Autodesk Inventor part; units mm, degrees
(part 4 of 5)
sketch "Sketch9" plane through (0, 0, -3) normal (0, 0, -1) x (-1, 0, 0)
  line L0 (143, 0.6) -> (143, 11.3716)
  line L1 (157, 15.8) -> (157, 15.2)
  line L2 (157, 15.2) -> (155.0929, 13.2929)
  line L3 (143.6142, 13) -> (154.3858, 13)
  line L4 (142.9071, 13.2929) -> (141, 15.2)
  line L5 (143.6142, 18) -> (154.3858, 18)
  line L6 (154.3858, 13) -> (143.6142, 13)
  line L7 (126.6142, 18) -> (137.3858, 18)
  line L8 (143, 11.3716) -> (143, 0.6)
  line L9 (138, 0.6) -> (138, 11.3716)
  line L10 (143, -5.6284) -> (143, -16.4)
  line L11 (138, -16.4) -> (138, -5.6284)
  line L12 (157, 15.8) -> (155.0929, 17.7071) projected
  line L13 (155.0929, 17.7071) -> (157, 15.8)
  line L14 (157, 15.2) -> (157, 15.8) projected
  line L15 (157, 15.8) -> (157, 15.2)
  line L16 (157, 15.2) -> (155.0929, 13.2929)
  line L17 (141, 15.8) -> (140, 15.8)
  line L18 (140, 15.8) -> (138.0929, 17.7071)
  line L19 (138.0929, 17.7071) -> (140, 15.8) projected
  line L20 (140.2, 13.9858) -> (140.2, 15.2)
  line L21 (140.2, 15.2) -> (140, 15.2)
  line L22 (138.2929, 12.0787) -> (140.2, 13.9858)
  line L23 (140.2, -2.0142) -> (138.2929, -0.1071) projected
  line L24 (138.2929, -0.1071) -> (140.2, -2.0142)
  line L25 (140.2, -2.0142) -> (140.2, -3.0142)
  line L26 (140.2, -3.0142) -> (138.2929, -4.9213)
  line L27 (138.2929, -17.1071) -> (140.2, -19.0142)
  line L28 (140.2, -19.0142) -> (140.8, -19.0142)
  line L29 (143, -16.4) -> (143, -5.6284)
  line L30 (140.8, -3.0142) -> (142.7071, -4.9213) projected
  line L31 (142.7071, -4.9213) -> (140.8, -3.0142)
  line L32 (140.8, -3.0142) -> (140.8, -2.0142)
  line L33 (142.7071, -0.1071) -> (140.8, -2.0142)
  line L34 (142.7071, 12.0787) -> (140.8, 13.9858)
  line L35 (140.8, 15.2) -> (141, 15.2)
  line L36 (140.8, 15.2) -> (140.8, 13.9858)
  line L37 (111.2, 0.5) -> (109.2929, 2.4071) projected
  line L38 (111.8, 16.5) -> (113.7071, 14.5929) projected
  line L39 (113.7071, 14.5929) -> (111.8, 16.5)
  line L40 (111.8, 16.5) -> (111.2, 16.5) projected
  line L41 (111.8, 16.5) -> (111.2, 16.5)
  line L42 (111.2, 16.5) -> (109.2929, 14.5929)
  line L43 (94.5, -0.2) -> (96.4071, 1.7071) projected
  line L44 (96.4071, 1.7071) -> (94.5, -0.2)
  line L45 (94.5, -0.2) -> (94.5, -0.8) projected
  line L46 (94.5, -0.2) -> (94.5, -0.8)
  line L47 (94.5, -0.8) -> (96.4071, -2.7071)
  line L48 (109.2929, -15.5929) -> (111.2, -17.5) projected
  line L49 (109.2929, -15.5929) -> (111.2, -17.5)
  line L50 (111.8, -17.5) -> (111.2, -17.5) projected
  line L51 (111.2, -17.5) -> (111.8, -17.5)
  line L52 (111.8, -17.5) -> (113.7071, -15.5929)
  line L53 (126.5929, -2.7071) -> (128.5, -0.8)
  line L54 (128.5, -0.2) -> (126.5929, 1.7071)
  line L55 (140.8, -19.0142) -> (140.2, -19.0142) projected
  line L56 (140.8, -19.0142) -> (142.7071, -17.1071)
  line L57 (140, 15.2) -> (138.0929, 13.2929)
  line L58 (125.9071, 13.2929) -> (124, 15.2)
  line L59 (124, 15.2) -> (124, 15.8)
  line L60 (124, 15.8) -> (125.9071, 17.7071)
  line L61 (126.6142, 18) -> (137.3858, 18)
  line L62 (126.6142, 13) -> (137.3858, 13)
  line L63 (110.5, -0.2) -> (108.75, 1.55)
  line L64 (108.5929, 1.7071) -> (110.5, -0.2) projected
  line L65 (108.5929, -2.7071) -> (110.5, -0.8) projected
  line L66 (110.5, -0.8) -> (108.5929, -2.7071)
  line L67 (110.5, -0.2) -> (108.5929, 1.7071)
  line L68 (113.7071, 2.4071) -> (111.8, 0.5) projected
  line L69 (111.8, 0.5) -> (113.7071, 2.4071)
  line L70 (112.5, -0.2) -> (114.4071, 1.7071) projected
  line L71 (112.5, -0.2) -> (114.4071, 1.7071)
  line L72 (112.5, -0.8) -> (114.4071, -2.7071)
  line L73 (109.2929, -3.4071) -> (111.2, -1.5) projected
  line L74 (111.2, -1.5) -> (109.2929, -3.4071)
  line L75 (111.8, -1.5) -> (113.7071, -3.4071)
  line L76 (113.7071, -3.4071) -> (111.8, -1.5) projected
  line L77 (111.2, 0.5) -> (109.2929, 2.4071)
  line L78 (111.2, -1.5) -> (111.2, -0.8)
  line L79 (111.2, -0.2) -> (111.2, 0.5)
  line L80 (110.5, -0.2) -> (111.2, -0.2)
  line L81 (111.8, -0.2) -> (112.5, -0.2)
  line L82 (111.8, 0.5) -> (111.8, -0.2)
  line L83 (111.8, -0.8) -> (111.8, -1.5)
  line L84 (112.5, -0.8) -> (111.8, -0.8)
  line L85 (111.2, -0.8) -> (110.5, -0.8)
  line L86 (97.1142, 2) -> (107.8858, 2)
  line L87 (109, 3.1142) -> (109, 13.8858)
  line L88 (109, -14.8858) -> (109, -4.1142)
  line L89 (107.8858, -3) -> (97.1142, -3)
  line L90 (114, -4.1142) -> (114, -14.8858)
  line L91 (125.8858, -3) -> (115.1142, -3)
  line L92 (114, 13.8858) -> (114, 3.1142)
  line L93 (115.1142, 2) -> (125.8858, 2)
  line L94 (-140, -35) -> (140, -35) projected
  line L95 (141, 15.8) -> (142.9071, 17.7071)
  line L96 (128.5, -0.2) -> (128.5, -0.8)
  line L97 (63.7142, 27) -> (80.4858, 27) projected
  line L98 (26.4142, 27) -> (43.1858, 27) projected
  line L99 (-20.3858, 27) -> (-3.6142, 27) projected
  line L100 (-57.6858, 27) -> (-40.9142, 27) projected
  line L101 (-104.4858, 27) -> (-87.7142, 27) projected
  line L102 (-141.7858, 27) -> (-125.0142, 27) projected
  line L103 (87, 20.4858) -> (87, 3.7142) projected
  line L104 (49.7, 20.4858) -> (49.7, 3.7142) projected
  line L105 (2.9, 20.4858) -> (2.9, 3.7142) projected
  line L106 (-34.4, 20.4858) -> (-34.4, 3.7142) projected
  line L107 (-81.2, 20.4858) -> (-81.2, 3.7142) projected
  line L108 (-118.5, 20.4858) -> (-118.5, 3.7142) projected
  line L109 (8.9, 9) -> (10.9, 11) projected
  line L110 (11.9, 11) -> (13.9, 9) projected
  line L111 (11.9, -9) -> (13.9, -11) projected
  line L112 (8.9, -11) -> (10.9, -9) projected
  line L113 (-72.2, 11) -> (-70.2, 9) projected
  line L114 (-70.2, 8) -> (-72.2, 6) projected
  line L115 (-72.2, -9) -> (-70.2, -11) projected
  line L116 (-75.2, -11) -> (-73.2, -9) projected
  arc A0 (109.2929, 14.5929) -> (109, 13.8858) centre (110, 13.8858) ccw
  arc A1 (114, 13.8858) -> (113.7071, 14.5929) centre (113, 13.8858) ccw
  arc A2 (113.7071, 2.4071) -> (114, 3.1142) centre (113, 3.1142) ccw
  arc A3 (109, 3.1142) -> (109.2929, 2.4071) centre (110, 3.1142) ccw
  arc A4 (108.5929, 1.7071) -> (107.8858, 2) centre (107.8858, 1) ccw
  arc A5 (115.1142, 2) -> (114.4071, 1.7071) centre (115.1142, 1) ccw
  arc A6 (114.4071, -2.7071) -> (115.1142, -3) centre (115.1142, -2) ccw
  arc A7 (114, -4.1142) -> (113.7071, -3.4071) centre (113, -4.1142) ccw
  arc A8 (109.2929, -3.4071) -> (109, -4.1142) centre (110, -4.1142) ccw
  arc A9 (107.8858, -3) -> (108.5929, -2.7071) centre (107.8858, -2) ccw
  arc A10 (97.1142, 2) -> (96.4071, 1.7071) centre (97.1142, 1) ccw
  arc A11 (96.4071, -2.7071) -> (97.1142, -3) centre (97.1142, -2) ccw
  arc A12 (109, -14.8858) -> (109.2929, -15.5929) centre (110, -14.8858) ccw
  arc A13 (113.7071, -15.5929) -> (114, -14.8858) centre (113, -14.8858) ccw
  arc A14 (125.8858, -3) -> (126.5929, -2.7071) centre (125.8858, -2) ccw
  arc A15 (126.5929, 1.7071) -> (125.8858, 2) centre (125.8858, 1) ccw
  arc A16 (138.0929, 17.7071) -> (137.3858, 18) centre (137.3858, 17) ccw
  arc A17 (126.6142, 18) -> (125.9071, 17.7071) centre (126.6142, 17) ccw
  arc A18 (125.9071, 13.2929) -> (126.6142, 13) centre (126.6142, 14) ccw
  arc A19 (137.3858, 13) -> (138.0929, 13.2929) centre (137.3858, 14) ccw
  arc A20 (138.2929, 12.0787) -> (138, 11.3716) centre (139, 11.3716) ccw
  arc A21 (143, 11.3716) -> (142.7071, 12.0787) centre (142, 11.3716) ccw
  arc A22 (142.9071, 13.2929) -> (143.6142, 13) centre (143.6142, 14) ccw
  arc A23 (143.6142, 18) -> (142.9071, 17.7071) centre (143.6142, 17) ccw
  arc A24 (155.0929, 17.7071) -> (154.3858, 18) centre (154.3858, 17) ccw
  arc A25 (154.3858, 13) -> (155.0929, 13.2929) centre (154.3858, 14) ccw
  arc A26 (154.3858, 13) -> (155.0929, 13.2929) centre (154.3858, 14) ccw
  arc A27 (138, 0.6) -> (138.2929, -0.1071) centre (139, 0.6) ccw
  arc A28 (142.7071, -0.1071) -> (143, 0.6) centre (142, 0.6) ccw
  arc A29 (143, -5.6284) -> (142.7071, -4.9213) centre (142, -5.6284) ccw
  arc A30 (138.2929, -4.9213) -> (138, -5.6284) centre (139, -5.6284) ccw
  arc A31 (138, -16.4) -> (138.2929, -17.1071) centre (139, -16.4) ccw
  arc A32 (142.7071, -17.1071) -> (143, -16.4) centre (142, -16.4) ccw
  line L117 (-58.3929, 1.9071) -> (-60.3, 0)
  line L118 (-39.1071, 3.0071) -> (-37.2, 1.1)
  line L119 (-38.3, 0) -> (-40.2071, 1.9071)
  line L120 (-40.2071, -2.5071) -> (-38.3, -0.6)
  line L121 (-38.3, -0.6) -> (-38.3, 0)
  line L122 (-38.3, 0) -> (-40.5, 2.2)
  line L123 (-40.2071, -22.8929) -> (-38.3, -24.8)
  line L124 (-39.1071, -21.7929) -> (-37.2, -23.7)
  line L125 (-59.4929, -21.7929) -> (-61.4, -23.7)
  line L126 (-58.3929, -22.8929) -> (-60.3, -24.8)
  line L127 (-38.3, 24.2) -> (-38.3, 24.8)
  line L128 (-58.3929, 26.7071) -> (-60.3, 24.8)
  line L129 (-60.3, 24.8) -> (-60.3, 24.2)
  line L130 (-60.3, 24.2) -> (-60.3, 24.8)
  line L131 (-58.3929, 22.2929) -> (-60.3, 24.2)
  line L132 (-59.4929, 21.1929) -> (-61.4, 23.1)
  line L133 (-62, 23.1) -> (-63.9071, 21.1929)
  line L134 (-63.9071, 3.0071) -> (-62, 1.1)
  line L135 (-62, 1.1) -> (-61.4, 1.1)
  line L136 (-61.4, 1.1) -> (-59.4929, 3.0071)
  line L137 (-59.4929, -3.6071) -> (-61.4, -1.7)
  line L138 (-62, -1.7) -> (-63.9071, -3.6071)
  line L139 (-64.2, -4.3142) -> (-64.2, -21.0858)
  line L140 (-63.9071, -21.7929) -> (-62, -23.7)
  line L141 (-60.3, -24.8) -> (-60.3, -25.4)
  line L142 (-60.3, -25.4) -> (-58.3929, -27.3071)
  line L143 (-57.6858, -27.6) -> (-40.9142, -27.6)
  line L144 (-40.2071, -27.3071) -> (-38.3, -25.4)
  line L145 (-38.3, -25.4) -> (-38.3, -24.8)
  line L146 (-37.2, -23.7) -> (-36.6, -23.7)
  line L147 (-36.6, -23.7) -> (-34.6929, -21.7929)
  line L148 (-34.4, -21.0858) -> (-34.4, -4.3142)
  line L149 (-34.6929, -3.6071) -> (-36.6, -1.7)
  line L150 (-36.6, -1.7) -> (-37.2, -1.7)
  line L151 (-37.2, -1.7) -> (-39.1071, -3.6071)
  line L152 (-38.3, -0.6) -> (-38.3, 0)
  line L153 (-36.6, 1.1) -> (-34.6929, 3.0071)
  line L154 (-34.4, 3.7142) -> (-34.4, 20.4858)
  line L155 (-34.6929, 21.1929) -> (-36.6, 23.1)
  line L156 (-36.6, 23.1) -> (-37.2, 23.1)
  line L157 (-37.2, 23.1) -> (-39.1071, 21.1929)
  line L158 (-38.3, 24.2) -> (-38.3, 24.8)
  line L159 (-57.6858, 27) -> (-40.9142, 27)
  line L160 (-64.2, 20.4858) -> (-64.2, 3.7142)
  line L161 (-38.3, 24.8) -> (-40.2071, 26.7071)
  line L162 (-38.3, 24.2) -> (-40.2071, 22.2929)
  line L163 (-37.2, 1.1) -> (-36.6, 1.1)
  arc A33 (-63.9071, 21.1929) -> (-64.2, 20.4858) centre (-63.2, 20.4858) ccw
  arc A34 (-57.6858, 27) -> (-58.3929, 26.7071) centre (-57.6858, 26) ccw
  arc A35 (-40.2071, 26.7071) -> (-40.9142, 27) centre (-40.9142, 26) ccw
  arc A36 (-34.4, 20.4858) -> (-34.6929, 21.1929) centre (-35.4, 20.4858) ccw
  arc A37 (-34.6929, 3.0071) -> (-34.4, 3.7142) centre (-35.4, 3.7142) ccw
  arc A38 (-34.4, -4.3142) -> (-34.6929, -3.6071) centre (-35.4, -4.3142) ccw
  arc A39 (-34.6929, -21.7929) -> (-34.4, -21.0858) centre (-35.4, -21.0858) ccw
  arc A40 (-40.9142, -27.6) -> (-40.2071, -27.3071) centre (-40.9142, -26.6) ccw
  arc A41 (-58.3929, -27.3071) -> (-57.6858, -27.6) centre (-57.6858, -26.6) ccw
  arc A42 (-64.2, -21.0858) -> (-63.9071, -21.7929) centre (-63.2, -21.0858) ccw
  arc A43 (-63.9071, -3.6071) -> (-64.2, -4.3142) centre (-63.2, -4.3142) ccw
  arc A44 (-64.2, 3.7142) -> (-63.9071, 3.0071) centre (-63.2, 3.7142) ccw
  line L164 (-62, 23.1) -> (-61.4, 23.1)
  line L165 (-60.3, 0) -> (-60.3, -0.6)
  line L166 (-58.3929, -2.5071) -> (-60.3, -0.6)
  line L167 (-62, -1.7) -> (-61.4, -1.7)
  line L168 (-62, -23.7) -> (-61.4, -23.7)
  line L169 (-57.1, 20.9) -> (-41.5, 20.9)
  line L170 (-39.4, 20.4858) -> (-39.4, 3.7142)
  line L171 (-41.5, 3.3) -> (-57.1, 3.3)
  line L172 (-59.2, 3.7142) -> (-59.2, 20.4858)
  line L173 (-57.6858, 22) -> (-40.9142, 22)
  line L174 (-40.5, 19.9) -> (-40.5, 4.3)
  line L175 (-40.9142, 2.2) -> (-57.6858, 2.2)
  line L176 (-58.1, 4.3) -> (-58.1, 19.9)
  line L177 (-57.1, -3.9) -> (-41.5, -3.9)
  line L178 (-39.4, -4.3142) -> (-39.4, -21.0858)
  line L179 (-41.5, -21.5) -> (-57.1, -21.5)
  line L180 (-59.2, -21.0858) -> (-59.2, -4.3142)
  line L181 (-57.6858, -22.6) -> (-40.9142, -22.6)
  line L182 (-40.5, -20.5) -> (-40.5, -4.9)
  line L183 (-40.9142, -2.8) -> (-57.6858, -2.8)
  line L184 (-58.1, -4.9) -> (-58.1, -20.5)
  arc A45 (-39.1071, 21.1929) -> (-39.4, 20.4858) centre (-38.4, 20.4858) ccw
  arc A46 (-40.9142, 22) -> (-40.2071, 22.2929) centre (-40.9142, 23) ccw
  arc A47 (-58.3929, 22.2929) -> (-57.6858, 22) centre (-57.6858, 23) ccw
  arc A48 (-59.2, 20.4858) -> (-59.4929, 21.1929) centre (-60.2, 20.4858) ccw
  arc A49 (-39.4, 3.7142) -> (-39.1071, 3.0071) centre (-38.4, 3.7142) ccw
  arc A50 (-39.1071, -3.6071) -> (-39.4, -4.3142) centre (-38.4, -4.3142) ccw
  arc A51 (-40.2071, 1.9071) -> (-40.9142, 2.2) centre (-40.9142, 1.2) ccw
  arc A52 (-40.9142, -2.8) -> (-40.2071, -2.5071) centre (-40.9142, -1.8) ccw
  arc A53 (-58.3929, -2.5071) -> (-57.6858, -2.8) centre (-57.6858, -1.8) ccw
  arc A54 (-57.6858, 2.2) -> (-58.3929, 1.9071) centre (-57.6858, 1.2) ccw
  arc A55 (-59.2, -4.3142) -> (-59.4929, -3.6071) centre (-60.2, -4.3142) ccw
  arc A56 (-59.4929, 3.0071) -> (-59.2, 3.7142) centre (-60.2, 3.7142) ccw
  arc A57 (-57.1, -3.9) -> (-58.1, -4.9) centre (-57.1, -4.9) ccw
  arc A58 (-40.5, -4.9) -> (-41.5, -3.9) centre (-41.5, -4.9) ccw
  arc A59 (-41.5, -21.5) -> (-40.5, -20.5) centre (-41.5, -20.5) ccw
  arc A60 (-40.2071, -22.8929) -> (-40.9142, -22.6) centre (-40.9142, -23.6) ccw
  arc A61 (-58.1, -20.5) -> (-57.1, -21.5) centre (-57.1, -20.5) ccw
  arc A62 (-59.4929, -21.7929) -> (-59.2, -21.0858) centre (-60.2, -21.0858) ccw
  arc A63 (-57.6858, -22.6) -> (-58.3929, -22.8929) centre (-57.6858, -23.6) ccw
  arc A64 (-40.5, 19.9) -> (-41.5, 20.9) centre (-41.5, 19.9) ccw
  arc A65 (-57.1, 20.9) -> (-58.1, 19.9) centre (-57.1, 19.9) ccw
  arc A66 (-41.5, 3.3) -> (-40.5, 4.3) centre (-41.5, 4.3) ccw
  arc A67 (-58.1, 4.3) -> (-57.1, 3.3) centre (-57.1, 4.3) ccw
  arc A68 (-39.4, -21.0858) -> (-39.1071, -21.7929) centre (-38.4, -21.0858) ccw
  line L185 (25.7071, 1.9071) -> (23.8, 0)
  line L186 (44.9929, 3.0071) -> (46.9, 1.1)
  line L187 (45.8, 0) -> (43.8929, 1.9071)
  line L188 (43.8929, -2.5071) -> (45.8, -0.6)
  line L189 (45.8, -0.6) -> (45.8, 0)
  line L190 (45.8, 0) -> (43.6, 2.2)
  line L191 (43.8929, -22.8929) -> (45.8, -24.8)
  line L192 (44.9929, -21.7929) -> (46.9, -23.7)
  line L193 (24.6071, -21.7929) -> (22.7, -23.7)
  line L194 (25.7071, -22.8929) -> (23.8, -24.8)
  line L195 (45.8, 24.2) -> (45.8, 24.8)
  line L196 (25.7071, 26.7071) -> (23.8, 24.8)
  line L197 (23.8, 24.8) -> (23.8, 24.2)
  line L198 (23.8, 24.2) -> (23.8, 24.8)
  line L199 (25.7071, 22.2929) -> (23.8, 24.2)
  line L200 (24.6071, 21.1929) -> (22.7, 23.1)
  line L201 (22.1, 23.1) -> (20.1929, 21.1929)
  line L202 (20.1929, 3.0071) -> (22.1, 1.1)
  line L203 (22.1, 1.1) -> (22.7, 1.1)
  line L204 (22.7, 1.1) -> (24.6071, 3.0071)
  line L205 (24.6071, -3.6071) -> (22.7, -1.7)
  line L206 (22.1, -1.7) -> (20.1929, -3.6071)
  line L207 (19.9, -4.3142) -> (19.9, -21.0858)
  line L208 (20.1929, -21.7929) -> (22.1, -23.7)
  line L209 (23.8, -24.8) -> (23.8, -25.4)
  line L210 (23.8, -25.4) -> (25.7071, -27.3071)
  line L211 (26.4142, -27.6) -> (43.1858, -27.6)
  line L212 (43.8929, -27.3071) -> (45.8, -25.4)
  line L213 (45.8, -25.4) -> (45.8, -24.8)
  line L214 (46.9, -23.7) -> (47.5, -23.7)
  line L215 (47.5, -23.7) -> (49.4071, -21.7929)
  line L216 (49.7, -21.0858) -> (49.7, -4.3142)
  line L217 (49.4071, -3.6071) -> (47.5, -1.7)
  line L218 (47.5, -1.7) -> (46.9, -1.7)
  line L219 (46.9, -1.7) -> (44.9929, -3.6071)
  line L220 (45.8, -0.6) -> (45.8, 0)
  line L221 (47.5, 1.1) -> (49.4071, 3.0071)
  line L222 (49.7, 3.7142) -> (49.7, 20.4858)
  line L223 (49.4071, 21.1929) -> (47.5, 23.1)
  line L224 (47.5, 23.1) -> (46.9, 23.1)
  line L225 (46.9, 23.1) -> (44.9929, 21.1929)
  line L226 (45.8, 24.2) -> (45.8, 24.8)
  line L227 (26.4142, 27) -> (43.1858, 27)
  line L228 (19.9, 20.4858) -> (19.9, 3.7142)
  line L229 (45.8, 24.8) -> (43.8929, 26.7071)
  line L230 (45.8, 24.2) -> (43.8929, 22.2929)
  line L231 (46.9, 1.1) -> (47.5, 1.1)
  arc A69 (20.1929, 21.1929) -> (19.9, 20.4858) centre (20.9, 20.4858) ccw
  arc A70 (26.4142, 27) -> (25.7071, 26.7071) centre (26.4142, 26) ccw
  arc A71 (43.8929, 26.7071) -> (43.1858, 27) centre (43.1858, 26) ccw
  arc A72 (49.7, 20.4858) -> (49.4071, 21.1929) centre (48.7, 20.4858) ccw
  arc A73 (49.4071, 3.0071) -> (49.7, 3.7142) centre (48.7, 3.7142) ccw
  arc A74 (49.7, -4.3142) -> (49.4071, -3.6071) centre (48.7, -4.3142) ccw
  arc A75 (49.4071, -21.7929) -> (49.7, -21.0858) centre (48.7, -21.0858) ccw
  arc A76 (43.1858, -27.6) -> (43.8929, -27.3071) centre (43.1858, -26.6) ccw
  arc A77 (25.7071, -27.3071) -> (26.4142, -27.6) centre (26.4142, -26.6) ccw
  arc A78 (19.9, -21.0858) -> (20.1929, -21.7929) centre (20.9, -21.0858) ccw
  arc A79 (20.1929, -3.6071) -> (19.9, -4.3142) centre (20.9, -4.3142) ccw
  arc A80 (19.9, 3.7142) -> (20.1929, 3.0071) centre (20.9, 3.7142) ccw
  line L232 (22.1, 23.1) -> (22.7, 23.1)
  line L233 (23.8, 0) -> (23.8, -0.6)
  line L234 (25.7071, -2.5071) -> (23.8, -0.6)
  line L235 (22.1, -1.7) -> (22.7, -1.7)
  line L236 (22.1, -23.7) -> (22.7, -23.7)
  line L237 (27, 20.9) -> (42.6, 20.9)
  line L238 (44.7, 20.4858) -> (44.7, 3.7142)
  line L239 (42.6, 3.3) -> (27, 3.3)
  line L240 (24.9, 3.7142) -> (24.9, 20.4858)
  line L241 (26.4142, 22) -> (43.1858, 22)
  line L242 (43.6, 19.9) -> (43.6, 4.3)
  line L243 (43.1858, 2.2) -> (26.4142, 2.2)
  line L244 (26, 4.3) -> (26, 19.9)
  line L245 (27, -3.9) -> (42.6, -3.9)
  line L246 (44.7, -4.3142) -> (44.7, -21.0858)
  line L247 (42.6, -21.5) -> (27, -21.5)
  line L248 (24.9, -21.0858) -> (24.9, -4.3142)
  line L249 (26.4142, -22.6) -> (43.1858, -22.6)
  line L250 (43.6, -20.5) -> (43.6, -4.9)
  line L251 (43.1858, -2.8) -> (26.4142, -2.8)
  line L252 (26, -4.9) -> (26, -20.5)
  arc A81 (44.9929, 21.1929) -> (44.7, 20.4858) centre (45.7, 20.4858) ccw
  arc A82 (43.1858, 22) -> (43.8929, 22.2929) centre (43.1858, 23) ccw
  arc A83 (25.7071, 22.2929) -> (26.4142, 22) centre (26.4142, 23) ccw
  arc A84 (24.9, 20.4858) -> (24.6071, 21.1929) centre (23.9, 20.4858) ccw
  arc A85 (44.7, 3.7142) -> (44.9929, 3.0071) centre (45.7, 3.7142) ccw
  arc A86 (44.9929, -3.6071) -> (44.7, -4.3142) centre (45.7, -4.3142) ccw
  arc A87 (43.8929, 1.9071) -> (43.1858, 2.2) centre (43.1858, 1.2) ccw
  arc A88 (43.1858, -2.8) -> (43.8929, -2.5071) centre (43.1858, -1.8) ccw
  arc A89 (25.7071, -2.5071) -> (26.4142, -2.8) centre (26.4142, -1.8) ccw
  arc A90 (26.4142, 2.2) -> (25.7071, 1.9071) centre (26.4142, 1.2) ccw
  arc A91 (24.9, -4.3142) -> (24.6071, -3.6071) centre (23.9, -4.3142) ccw
  arc A92 (24.6071, 3.0071) -> (24.9, 3.7142) centre (23.9, 3.7142) ccw
  arc A93 (27, -3.9) -> (26, -4.9) centre (27, -4.9) ccw
  arc A94 (43.6, -4.9) -> (42.6, -3.9) centre (42.6, -4.9) ccw
  arc A95 (42.6, -21.5) -> (43.6, -20.5) centre (42.6, -20.5) ccw
  arc A96 (43.8929, -22.8929) -> (43.1858, -22.6) centre (43.1858, -23.6) ccw
  arc A97 (26, -20.5) -> (27, -21.5) centre (27, -20.5) ccw
  arc A98 (24.6071, -21.7929) -> (24.9, -21.0858) centre (23.9, -21.0858) ccw
  arc A99 (26.4142, -22.6) -> (25.7071, -22.8929) centre (26.4142, -23.6) ccw
  arc A100 (43.6, 19.9) -> (42.6, 20.9) centre (42.6, 19.9) ccw
  arc A101 (27, 20.9) -> (26, 19.9) centre (27, 19.9) ccw
  arc A102 (42.6, 3.3) -> (43.6, 4.3) centre (42.6, 4.3) ccw
  arc A103 (26, 4.3) -> (27, 3.3) centre (27, 4.3) ccw
  arc A104 (44.7, -21.0858) -> (44.9929, -21.7929) centre (45.7, -21.0858) ccw
  line L253 (-21.0929, 1.9071) -> (-23, 0)
  line L254 (-1.8071, 3.0071) -> (0.1, 1.1)
  line L255 (-1, 0) -> (-2.9071, 1.9071)
  line L256 (-2.9071, -2.5071) -> (-1, -0.6)
  line L257 (-1, -0.6) -> (-1, 0)
  line L258 (-1, 0) -> (-3.2, 2.2)
  line L259 (-2.9071, -22.8929) -> (-1, -24.8)
  line L260 (-1.8071, -21.7929) -> (0.1, -23.7)
  line L261 (-22.1929, -21.7929) -> (-24.1, -23.7)
  line L262 (-21.0929, -22.8929) -> (-23, -24.8)
  line L263 (-1, 24.2) -> (-1, 24.8)
  line L264 (-21.0929, 26.7071) -> (-23, 24.8)
  line L265 (-23, 24.8) -> (-23, 24.2)
  line L266 (-23, 24.2) -> (-23, 24.8)
  line L267 (-21.0929, 22.2929) -> (-23, 24.2)
  line L268 (-22.1929, 21.1929) -> (-24.1, 23.1)
  line L269 (-24.7, 23.1) -> (-26.6071, 21.1929)
  line L270 (-26.6071, 3.0071) -> (-24.7, 1.1)
  line L271 (-24.7, 1.1) -> (-24.1, 1.1)
  line L272 (-24.1, 1.1) -> (-22.1929, 3.0071)
  line L273 (-22.1929, -3.6071) -> (-24.1, -1.7)
  line L274 (-24.7, -1.7) -> (-26.6071, -3.6071)
  line L275 (-26.9, -4.3142) -> (-26.9, -21.0858)
  line L276 (-26.6071, -21.7929) -> (-24.7, -23.7)
  line L277 (-23, -24.8) -> (-23, -25.4)
  line L278 (-23, -25.4) -> (-21.0929, -27.3071)
  line L279 (-20.3858, -27.6) -> (-3.6142, -27.6)
  line L280 (-2.9071, -27.3071) -> (-1, -25.4)
  line L281 (-1, -25.4) -> (-1, -24.8)
  line L282 (0.1, -23.7) -> (0.7, -23.7)
  line L283 (0.7, -23.7) -> (2.6071, -21.7929)
  line L284 (2.9, -21.0858) -> (2.9, -4.3142)
  line L285 (2.6071, -3.6071) -> (0.7, -1.7)
  line L286 (0.7, -1.7) -> (0.1, -1.7)
  line L287 (0.1, -1.7) -> (-1.8071, -3.6071)
  line L288 (-1, -0.6) -> (-1, 0)
  line L289 (0.7, 1.1) -> (2.6071, 3.0071)
  line L290 (2.9, 3.7142) -> (2.9, 20.4858)
  line L291 (2.6071, 21.1929) -> (0.7, 23.1)
  line L292 (0.7, 23.1) -> (0.1, 23.1)
  line L293 (0.1, 23.1) -> (-1.8071, 21.1929)
  line L294 (-1, 24.2) -> (-1, 24.8)
  line L295 (-20.3858, 27) -> (-3.6142, 27)
  line L296 (-26.9, 20.4858) -> (-26.9, 3.7142)
  line L297 (-1, 24.8) -> (-2.9071, 26.7071)
  line L298 (-1, 24.2) -> (-2.9071, 22.2929)
  line L299 (0.1, 1.1) -> (0.7, 1.1)
  arc A105 (-26.6071, 21.1929) -> (-26.9, 20.4858) centre (-25.9, 20.4858) ccw
  arc A106 (-20.3858, 27) -> (-21.0929, 26.7071) centre (-20.3858, 26) ccw
  arc A107 (-2.9071, 26.7071) -> (-3.6142, 27) centre (-3.6142, 26) ccw
  arc A108 (2.9, 20.4858) -> (2.6071, 21.1929) centre (1.9, 20.4858) ccw
  arc A109 (2.6071, 3.0071) -> (2.9, 3.7142) centre (1.9, 3.7142) ccw
  arc A110 (2.9, -4.3142) -> (2.6071, -3.6071) centre (1.9, -4.3142) ccw
  arc A111 (2.6071, -21.7929) -> (2.9, -21.0858) centre (1.9, -21.0858) ccw
  arc A112 (-3.6142, -27.6) -> (-2.9071, -27.3071) centre (-3.6142, -26.6) ccw
  arc A113 (-21.0929, -27.3071) -> (-20.3858, -27.6) centre (-20.3858, -26.6) ccw
  arc A114 (-26.9, -21.0858) -> (-26.6071, -21.7929) centre (-25.9, -21.0858) ccw
  arc A115 (-26.6071, -3.6071) -> (-26.9, -4.3142) centre (-25.9, -4.3142) ccw
  arc A116 (-26.9, 3.7142) -> (-26.6071, 3.0071) centre (-25.9, 3.7142) ccw
  line L300 (-24.7, 23.1) -> (-24.1, 23.1)
  line L301 (-23, 0) -> (-23, -0.6)
  line L302 (-21.0929, -2.5071) -> (-23, -0.6)
  line L303 (-24.7, -1.7) -> (-24.1, -1.7)
  line L304 (-24.7, -23.7) -> (-24.1, -23.7)
  line L305 (-19.8, 20.9) -> (-4.2, 20.9)
  line L306 (-2.1, 20.4858) -> (-2.1, 3.7142)
  line L307 (-4.2, 3.3) -> (-19.8, 3.3)
  line L308 (-21.9, 3.7142) -> (-21.9, 20.4858)
  line L309 (-20.3858, 22) -> (-3.6142, 22)
  line L310 (-3.2, 19.9) -> (-3.2, 4.3)
  line L311 (-3.6142, 2.2) -> (-20.3858, 2.2)
  line L312 (-20.8, 4.3) -> (-20.8, 19.9)
  line L313 (-19.8, -3.9) -> (-4.2, -3.9)
  line L314 (-2.1, -4.3142) -> (-2.1, -21.0858)
  line L315 (-4.2, -21.5) -> (-19.8, -21.5)
  line L316 (-21.9, -21.0858) -> (-21.9, -4.3142)
  line L317 (-20.3858, -22.6) -> (-3.6142, -22.6)
  line L318 (-3.2, -20.5) -> (-3.2, -4.9)
  line L319 (-3.6142, -2.8) -> (-20.3858, -2.8)
  line L320 (-20.8, -4.9) -> (-20.8, -20.5)
  arc A117 (-1.8071, 21.1929) -> (-2.1, 20.4858) centre (-1.1, 20.4858) ccw
  arc A118 (-3.6142, 22) -> (-2.9071, 22.2929) centre (-3.6142, 23) ccw
  arc A119 (-21.0929, 22.2929) -> (-20.3858, 22) centre (-20.3858, 23) ccw
  arc A120 (-21.9, 20.4858) -> (-22.1929, 21.1929) centre (-22.9, 20.4858) ccw
  arc A121 (-2.1, 3.7142) -> (-1.8071, 3.0071) centre (-1.1, 3.7142) ccw
  arc A122 (-1.8071, -3.6071) -> (-2.1, -4.3142) centre (-1.1, -4.3142) ccw
  arc A123 (-2.9071, 1.9071) -> (-3.6142, 2.2) centre (-3.6142, 1.2) ccw
  arc A124 (-3.6142, -2.8) -> (-2.9071, -2.5071) centre (-3.6142, -1.8) ccw
  arc A125 (-21.0929, -2.5071) -> (-20.3858, -2.8) centre (-20.3858, -1.8) ccw
  arc A126 (-20.3858, 2.2) -> (-21.0929, 1.9071) centre (-20.3858, 1.2) ccw
  arc A127 (-21.9, -4.3142) -> (-22.1929, -3.6071) centre (-22.9, -4.3142) ccw
  arc A128 (-22.1929, 3.0071) -> (-21.9, 3.7142) centre (-22.9, 3.7142) ccw
  arc A129 (-19.8, -3.9) -> (-20.8, -4.9) centre (-19.8, -4.9) ccw
  arc A130 (-3.2, -4.9) -> (-4.2, -3.9) centre (-4.2, -4.9) ccw
  arc A131 (-4.2, -21.5) -> (-3.2, -20.5) centre (-4.2, -20.5) ccw
  arc A132 (-2.9071, -22.8929) -> (-3.6142, -22.6) centre (-3.6142, -23.6) ccw
  arc A133 (-20.8, -20.5) -> (-19.8, -21.5) centre (-19.8, -20.5) ccw
  arc A134 (-22.1929, -21.7929) -> (-21.9, -21.0858) centre (-22.9, -21.0858) ccw
  arc A135 (-20.3858, -22.6) -> (-21.0929, -22.8929) centre (-20.3858, -23.6) ccw
  arc A136 (-3.2, 19.9) -> (-4.2, 20.9) centre (-4.2, 19.9) ccw
  arc A137 (-19.8, 20.9) -> (-20.8, 19.9) centre (-19.8, 19.9) ccw
  arc A138 (-4.2, 3.3) -> (-3.2, 4.3) centre (-4.2, 4.3) ccw
  arc A139 (-20.8, 4.3) -> (-19.8, 3.3) centre (-19.8, 4.3) ccw
  arc A140 (-2.1, -21.0858) -> (-1.8071, -21.7929) centre (-1.1, -21.0858) ccw
  line L321 (63.0071, 1.9071) -> (61.1, 0)
  line L322 (82.2929, 3.0071) -> (84.2, 1.1)
  line L323 (83.1, 0) -> (81.1929, 1.9071)
  line L324 (81.1929, -2.5071) -> (83.1, -0.6)
  line L325 (83.1, -0.6) -> (83.1, 0)
  line L326 (83.1, 0) -> (80.9, 2.2)
  line L327 (81.1929, -22.8929) -> (83.1, -24.8)
  line L328 (82.2929, -21.7929) -> (84.2, -23.7)
  line L329 (61.9071, -21.7929) -> (60, -23.7)
  line L330 (63.0071, -22.8929) -> (61.1, -24.8)
  line L331 (83.1, 24.2) -> (83.1, 24.8)
  line L332 (63.0071, 26.7071) -> (61.1, 24.8)
  line L333 (61.1, 24.8) -> (61.1, 24.2)
  line L334 (61.1, 24.2) -> (61.1, 24.8)
  line L335 (63.0071, 22.2929) -> (61.1, 24.2)
  line L336 (61.9071, 21.1929) -> (60, 23.1)
  line L337 (59.4, 23.1) -> (57.4929, 21.1929)
  line L338 (57.4929, 3.0071) -> (59.4, 1.1)
  line L339 (59.4, 1.1) -> (60, 1.1)
  line L340 (60, 1.1) -> (61.9071, 3.0071)
  line L341 (61.9071, -3.6071) -> (60, -1.7)
  line L342 (59.4, -1.7) -> (57.4929, -3.6071)
  line L343 (57.2, -4.3142) -> (57.2, -21.0858)
  line L344 (57.4929, -21.7929) -> (59.4, -23.7)
  line L345 (61.1, -24.8) -> (61.1, -25.4)
  line L346 (61.1, -25.4) -> (63.0071, -27.3071)
  line L347 (63.7142, -27.6) -> (80.4858, -27.6)
  line L348 (81.1929, -27.3071) -> (83.1, -25.4)
  line L349 (83.1, -25.4) -> (83.1, -24.8)
  line L350 (84.2, -23.7) -> (84.8, -23.7)
  line L351 (84.8, -23.7) -> (86.7071, -21.7929)
  line L352 (87, -21.0858) -> (87, -4.3142)
  line L353 (86.7071, -3.6071) -> (84.8, -1.7)
  line L354 (84.8, -1.7) -> (84.2, -1.7)
  line L355 (84.2, -1.7) -> (82.2929, -3.6071)
  line L356 (83.1, -0.6) -> (83.1, 0)
  line L357 (84.8, 1.1) -> (86.7071, 3.0071)
  line L358 (87, 3.7142) -> (87, 20.4858)
  line L359 (86.7071, 21.1929) -> (84.8, 23.1)
  line L360 (84.8, 23.1) -> (84.2, 23.1)
  line L361 (84.2, 23.1) -> (82.2929, 21.1929)
  line L362 (83.1, 24.2) -> (83.1, 24.8)
  line L363 (63.7142, 27) -> (80.4858, 27)
  line L364 (57.2, 20.4858) -> (57.2, 3.7142)
  line L365 (83.1, 24.8) -> (81.1929, 26.7071)
  line L366 (83.1, 24.2) -> (81.1929, 22.2929)
  line L367 (84.2, 1.1) -> (84.8, 1.1)
  arc A141 (57.4929, 21.1929) -> (57.2, 20.4858) centre (58.2, 20.4858) ccw
  arc A142 (63.7142, 27) -> (63.0071, 26.7071) centre (63.7142, 26) ccw
  arc A143 (81.1929, 26.7071) -> (80.4858, 27) centre (80.4858, 26) ccw
  arc A144 (87, 20.4858) -> (86.7071, 21.1929) centre (86, 20.4858) ccw
  arc A145 (86.7071, 3.0071) -> (87, 3.7142) centre (86, 3.7142) ccw
  arc A146 (87, -4.3142) -> (86.7071, -3.6071) centre (86, -4.3142) ccw
  arc A147 (86.7071, -21.7929) -> (87, -21.0858) centre (86, -21.0858) ccw
  arc A148 (80.4858, -27.6) -> (81.1929, -27.3071) centre (80.4858, -26.6) ccw
  arc A149 (63.0071, -27.3071) -> (63.7142, -27.6) centre (63.7142, -26.6) ccw
  arc A150 (57.2, -21.0858) -> (57.4929, -21.7929) centre (58.2, -21.0858) ccw
  arc A151 (57.4929, -3.6071) -> (57.2, -4.3142) centre (58.2, -4.3142) ccw
  arc A152 (57.2, 3.7142) -> (57.4929, 3.0071) centre (58.2, 3.7142) ccw
  line L368 (59.4, 23.1) -> (60, 23.1)
  line L369 (61.1, 0) -> (61.1, -0.6)
  line L370 (63.0071, -2.5071) -> (61.1, -0.6)
  line L371 (59.4, -1.7) -> (60, -1.7)
  line L372 (59.4, -23.7) -> (60, -23.7)
  line L373 (64.3, 20.9) -> (79.9, 20.9)
  line L374 (82, 20.4858) -> (82, 3.7142)
  line L375 (79.9, 3.3) -> (64.3, 3.3)
  line L376 (62.2, 3.7142) -> (62.2, 20.4858)
  line L377 (63.7142, 22) -> (80.4858, 22)
  line L378 (80.9, 19.9) -> (80.9, 4.3)
  line L379 (80.4858, 2.2) -> (63.7142, 2.2)
  line L380 (63.3, 4.3) -> (63.3, 19.9)
  line L381 (64.3, -3.9) -> (79.9, -3.9)
  line L382 (82, -4.3142) -> (82, -21.0858)
  line L383 (79.9, -21.5) -> (64.3, -21.5)
  line L384 (62.2, -21.0858) -> (62.2, -4.3142)
  line L385 (63.7142, -22.6) -> (80.4858, -22.6)
  line L386 (80.9, -20.5) -> (80.9, -4.9)
  line L387 (80.4858, -2.8) -> (63.7142, -2.8)
  line L388 (63.3, -4.9) -> (63.3, -20.5)
  arc A153 (82.2929, 21.1929) -> (82, 20.4858) centre (83, 20.4858) ccw
  arc A154 (80.4858, 22) -> (81.1929, 22.2929) centre (80.4858, 23) ccw
  arc A155 (63.0071, 22.2929) -> (63.7142, 22) centre (63.7142, 23) ccw
  arc A156 (62.2, 20.4858) -> (61.9071, 21.1929) centre (61.2, 20.4858) ccw
  arc A157 (82, 3.7142) -> (82.2929, 3.0071) centre (83, 3.7142) ccw
  arc A158 (82.2929, -3.6071) -> (82, -4.3142) centre (83, -4.3142) ccw
  arc A159 (81.1929, 1.9071) -> (80.4858, 2.2) centre (80.4858, 1.2) ccw
  arc A160 (80.4858, -2.8) -> (81.1929, -2.5071) centre (80.4858, -1.8) ccw
  arc A161 (63.0071, -2.5071) -> (63.7142, -2.8) centre (63.7142, -1.8) ccw
  arc A162 (63.7142, 2.2) -> (63.0071, 1.9071) centre (63.7142, 1.2) ccw
  arc A163 (62.2, -4.3142) -> (61.9071, -3.6071) centre (61.2, -4.3142) ccw
  arc A164 (61.9071, 3.0071) -> (62.2, 3.7142) centre (61.2, 3.7142) ccw
  arc A165 (64.3, -3.9) -> (63.3, -4.9) centre (64.3, -4.9) ccw
  arc A166 (80.9, -4.9) -> (79.9, -3.9) centre (79.9, -4.9) ccw
  arc A167 (79.9, -21.5) -> (80.9, -20.5) centre (79.9, -20.5) ccw
  arc A168 (81.1929, -22.8929) -> (80.4858, -22.6) centre (80.4858, -23.6) ccw
  arc A169 (63.3, -20.5) -> (64.3, -21.5) centre (64.3, -20.5) ccw
  arc A170 (61.9071, -21.7929) -> (62.2, -21.0858) centre (61.2, -21.0858) ccw
  arc A171 (63.7142, -22.6) -> (63.0071, -22.8929) centre (63.7142, -23.6) ccw
  arc A172 (80.9, 19.9) -> (79.9, 20.9) centre (79.9, 19.9) ccw
  arc A173 (64.3, 20.9) -> (63.3, 19.9) centre (64.3, 19.9) ccw
  arc A174 (79.9, 3.3) -> (80.9, 4.3) centre (79.9, 4.3) ccw
  arc A175 (63.3, 4.3) -> (64.3, 3.3) centre (64.3, 4.3) ccw
  arc A176 (82, -21.0858) -> (82.2929, -21.7929) centre (83, -21.0858) ccw
  line L389 (-142.4929, 1.9071) -> (-144.4, 0)
  line L390 (-123.2071, 3.0071) -> (-121.3, 1.1)
  line L391 (-122.4, 0) -> (-124.3071, 1.9071)
  line L392 (-124.3071, -2.5071) -> (-122.4, -0.6)
  line L393 (-122.4, -0.6) -> (-122.4, 0)
  line L394 (-122.4, 0) -> (-124.6, 2.2)
  line L395 (-124.3071, -22.8929) -> (-122.4, -24.8)
  line L396 (-123.2071, -21.7929) -> (-121.3, -23.7)
  line L397 (-143.5929, -21.7929) -> (-145.5, -23.7)
  line L398 (-142.4929, -22.8929) -> (-144.4, -24.8)
  line L399 (-122.4, 24.2) -> (-122.4, 24.8)
  line L400 (-142.4929, 26.7071) -> (-144.4, 24.8)
  line L401 (-144.4, 24.8) -> (-144.4, 24.2)
  line L402 (-144.4, 24.2) -> (-144.4, 24.8)
  line L403 (-142.4929, 22.2929) -> (-144.4, 24.2)
  line L404 (-143.5929, 21.1929) -> (-145.5, 23.1)
  line L405 (-146.1, 23.1) -> (-148.0071, 21.1929)
  line L406 (-148.0071, 3.0071) -> (-146.1, 1.1)
  line L407 (-146.1, 1.1) -> (-145.5, 1.1)
  line L408 (-145.5, 1.1) -> (-143.5929, 3.0071)
  line L409 (-143.5929, -3.6071) -> (-145.5, -1.7)
  line L410 (-146.1, -1.7) -> (-148.0071, -3.6071)
  line L411 (-148.3, -4.3142) -> (-148.3, -21.0858)
  line L412 (-148.0071, -21.7929) -> (-146.1, -23.7)
  line L413 (-144.4, -24.8) -> (-144.4, -25.4)
  line L414 (-144.4, -25.4) -> (-142.4929, -27.3071)
  line L415 (-141.7858, -27.6) -> (-125.0142, -27.6)
  line L416 (-124.3071, -27.3071) -> (-122.4, -25.4)
  line L417 (-122.4, -25.4) -> (-122.4, -24.8)
  line L418 (-121.3, -23.7) -> (-120.7, -23.7)
  line L419 (-120.7, -23.7) -> (-118.7929, -21.7929)
  line L420 (-118.5, -21.0858) -> (-118.5, -4.3142)
  line L421 (-118.7929, -3.6071) -> (-120.7, -1.7)
  line L422 (-120.7, -1.7) -> (-121.3, -1.7)
  line L423 (-121.3, -1.7) -> (-123.2071, -3.6071)
  line L424 (-122.4, -0.6) -> (-122.4, 0)
  line L425 (-120.7, 1.1) -> (-118.7929, 3.0071)
  line L426 (-118.5, 3.7142) -> (-118.5, 20.4858)
  line L427 (-118.7929, 21.1929) -> (-120.7, 23.1)
  line L428 (-120.7, 23.1) -> (-121.3, 23.1)
  line L429 (-121.3, 23.1) -> (-123.2071, 21.1929)
  line L430 (-122.4, 24.2) -> (-122.4, 24.8)
  line L431 (-141.7858, 27) -> (-125.0142, 27)
  line L432 (-148.3, 20.4858) -> (-148.3, 3.7142)
  line L433 (-122.4, 24.8) -> (-124.3071, 26.7071)
  line L434 (-122.4, 24.2) -> (-124.3071, 22.2929)
  line L435 (-121.3, 1.1) -> (-120.7, 1.1)
  arc A177 (-148.0071, 21.1929) -> (-148.3, 20.4858) centre (-147.3, 20.4858) ccw
  arc A178 (-141.7858, 27) -> (-142.4929, 26.7071) centre (-141.7858, 26) ccw
  arc A179 (-124.3071, 26.7071) -> (-125.0142, 27) centre (-125.0142, 26) ccw
  arc A180 (-118.5, 20.4858) -> (-118.7929, 21.1929) centre (-119.5, 20.4858) ccw
  arc A181 (-118.7929, 3.0071) -> (-118.5, 3.7142) centre (-119.5, 3.7142) ccw
  arc A182 (-118.5, -4.3142) -> (-118.7929, -3.6071) centre (-119.5, -4.3142) ccw
  arc A183 (-118.7929, -21.7929) -> (-118.5, -21.0858) centre (-119.5, -21.0858) ccw
  arc A184 (-125.0142, -27.6) -> (-124.3071, -27.3071) centre (-125.0142, -26.6) ccw
  arc A185 (-142.4929, -27.3071) -> (-141.7858, -27.6) centre (-141.7858, -26.6) ccw
  arc A186 (-148.3, -21.0858) -> (-148.0071, -21.7929) centre (-147.3, -21.0858) ccw
  arc A187 (-148.0071, -3.6071) -> (-148.3, -4.3142) centre (-147.3, -4.3142) ccw
  arc A188 (-148.3, 3.7142) -> (-148.0071, 3.0071) centre (-147.3, 3.7142) ccw
  line L436 (-146.1, 23.1) -> (-145.5, 23.1)
  line L437 (-144.4, 0) -> (-144.4, -0.6)
  line L438 (-142.4929, -2.5071) -> (-144.4, -0.6)
  line L439 (-146.1, -1.7) -> (-145.5, -1.7)
  line L440 (-146.1, -23.7) -> (-145.5, -23.7)
  line L441 (-141.2, 20.9) -> (-125.6, 20.9)
  line L442 (-123.5, 20.4858) -> (-123.5, 3.7142)
  line L443 (-125.6, 3.3) -> (-141.2, 3.3)
  line L444 (-143.3, 3.7142) -> (-143.3, 20.4858)
  line L445 (-141.7858, 22) -> (-125.0142, 22)
  line L446 (-124.6, 19.9) -> (-124.6, 4.3)
  line L447 (-125.0142, 2.2) -> (-141.7858, 2.2)
  line L448 (-142.2, 4.3) -> (-142.2, 19.9)
  line L449 (-141.2, -3.9) -> (-125.6, -3.9)
  line L450 (-123.5, -4.3142) -> (-123.5, -21.0858)
  line L451 (-125.6, -21.5) -> (-141.2, -21.5)
  line L452 (-143.3, -21.0858) -> (-143.3, -4.3142)
  line L453 (-141.7858, -22.6) -> (-125.0142, -22.6)
  line L454 (-124.6, -20.5) -> (-124.6, -4.9)
  line L455 (-125.0142, -2.8) -> (-141.7858, -2.8)
  line L456 (-142.2, -4.9) -> (-142.2, -20.5)
  arc A189 (-123.2071, 21.1929) -> (-123.5, 20.4858) centre (-122.5, 20.4858) ccw
  arc A190 (-125.0142, 22) -> (-124.3071, 22.2929) centre (-125.0142, 23) ccw
  arc A191 (-142.4929, 22.2929) -> (-141.7858, 22) centre (-141.7858, 23) ccw
  arc A192 (-143.3, 20.4858) -> (-143.5929, 21.1929) centre (-144.3, 20.4858) ccw
  arc A193 (-123.5, 3.7142) -> (-123.2071, 3.0071) centre (-122.5, 3.7142) ccw
  arc A194 (-123.2071, -3.6071) -> (-123.5, -4.3142) centre (-122.5, -4.3142) ccw
  arc A195 (-124.3071, 1.9071) -> (-125.0142, 2.2) centre (-125.0142, 1.2) ccw
  arc A196 (-125.0142, -2.8) -> (-124.3071, -2.5071) centre (-125.0142, -1.8) ccw
  arc A197 (-142.4929, -2.5071) -> (-141.7858, -2.8) centre (-141.7858, -1.8) ccw
  arc A198 (-141.7858, 2.2) -> (-142.4929, 1.9071) centre (-141.7858, 1.2) ccw
  arc A199 (-143.3, -4.3142) -> (-143.5929, -3.6071) centre (-144.3, -4.3142) ccw
  arc A200 (-143.5929, 3.0071) -> (-143.3, 3.7142) centre (-144.3, 3.7142) ccw
  arc A201 (-141.2, -3.9) -> (-142.2, -4.9) centre (-141.2, -4.9) ccw
  arc A202 (-124.6, -4.9) -> (-125.6, -3.9) centre (-125.6, -4.9) ccw
  arc A203 (-125.6, -21.5) -> (-124.6, -20.5) centre (-125.6, -20.5) ccw
  arc A204 (-124.3071, -22.8929) -> (-125.0142, -22.6) centre (-125.0142, -23.6) ccw
  arc A205 (-142.2, -20.5) -> (-141.2, -21.5) centre (-141.2, -20.5) ccw
  arc A206 (-143.5929, -21.7929) -> (-143.3, -21.0858) centre (-144.3, -21.0858) ccw
  arc A207 (-141.7858, -22.6) -> (-142.4929, -22.8929) centre (-141.7858, -23.6) ccw
  arc A208 (-124.6, 19.9) -> (-125.6, 20.9) centre (-125.6, 19.9) ccw
  arc A209 (-141.2, 20.9) -> (-142.2, 19.9) centre (-141.2, 19.9) ccw
  arc A210 (-125.6, 3.3) -> (-124.6, 4.3) centre (-125.6, 4.3) ccw
  arc A211 (-142.2, 4.3) -> (-141.2, 3.3) centre (-141.2, 4.3) ccw
  arc A212 (-123.5, -21.0858) -> (-123.2071, -21.7929) centre (-122.5, -21.0858) ccw
  line L457 (-105.1929, 1.9071) -> (-107.1, 0)
  line L458 (-85.9071, 3.0071) -> (-84, 1.1)
  line L459 (-85.1, 0) -> (-87.0071, 1.9071)
  line L460 (-87.0071, -2.5071) -> (-85.1, -0.6)
  line L461 (-85.1, -0.6) -> (-85.1, 0)
  line L462 (-85.1, 0) -> (-87.3, 2.2)
  line L463 (-87.0071, -22.8929) -> (-85.1, -24.8)
  line L464 (-85.9071, -21.7929) -> (-84, -23.7)
  line L465 (-106.2929, -21.7929) -> (-108.2, -23.7)
  line L466 (-105.1929, -22.8929) -> (-107.1, -24.8)
  line L467 (-85.1, 24.2) -> (-85.1, 24.8)
  line L468 (-105.1929, 26.7071) -> (-107.1, 24.8)
  line L469 (-107.1, 24.8) -> (-107.1, 24.2)
  line L470 (-107.1, 24.2) -> (-107.1, 24.8)
  line L471 (-105.1929, 22.2929) -> (-107.1, 24.2)
  line L472 (-106.2929, 21.1929) -> (-108.2, 23.1)
  line L473 (-108.8, 23.1) -> (-110.7071, 21.1929)
  line L474 (-110.7071, 3.0071) -> (-108.8, 1.1)
  line L475 (-108.8, 1.1) -> (-108.2, 1.1)
  line L476 (-108.2, 1.1) -> (-106.2929, 3.0071)
  line L477 (-106.2929, -3.6071) -> (-108.2, -1.7)
  line L478 (-108.8, -1.7) -> (-110.7071, -3.6071)
  line L479 (-111, -4.3142) -> (-111, -21.0858)
  line L480 (-110.7071, -21.7929) -> (-108.8, -23.7)
  line L481 (-107.1, -24.8) -> (-107.1, -25.4)
  line L482 (-107.1, -25.4) -> (-105.1929, -27.3071)
  line L483 (-104.4858, -27.6) -> (-87.7142, -27.6)
  line L484 (-87.0071, -27.3071) -> (-85.1, -25.4)
  line L485 (-85.1, -25.4) -> (-85.1, -24.8)
  line L486 (-84, -23.7) -> (-83.4, -23.7)
  line L487 (-83.4, -23.7) -> (-81.4929, -21.7929)
  line L488 (-81.2, -21.0858) -> (-81.2, -4.3142)
  line L489 (-81.4929, -3.6071) -> (-83.4, -1.7)
  line L490 (-83.4, -1.7) -> (-84, -1.7)
  line L491 (-84, -1.7) -> (-85.9071, -3.6071)
  line L492 (-85.1, -0.6) -> (-85.1, 0)
  line L493 (-83.4, 1.1) -> (-81.4929, 3.0071)
  line L494 (-81.2, 3.7142) -> (-81.2, 20.4858)
  line L495 (-81.4929, 21.1929) -> (-83.4, 23.1)
  line L496 (-83.4, 23.1) -> (-84, 23.1)
  line L497 (-84, 23.1) -> (-85.9071, 21.1929)
  line L498 (-85.1, 24.2) -> (-85.1, 24.8)
  line L499 (-104.4858, 27) -> (-87.7142, 27)
  line L500 (-111, 20.4858) -> (-111, 3.7142)
  line L501 (-85.1, 24.8) -> (-87.0071, 26.7071)
  line L502 (-85.1, 24.2) -> (-87.0071, 22.2929)
  line L503 (-84, 1.1) -> (-83.4, 1.1)
  arc A213 (-110.7071, 21.1929) -> (-111, 20.4858) centre (-110, 20.4858) ccw
  arc A214 (-104.4858, 27) -> (-105.1929, 26.7071) centre (-104.4858, 26) ccw
  arc A215 (-87.0071, 26.7071) -> (-87.7142, 27) centre (-87.7142, 26) ccw
  arc A216 (-81.2, 20.4858) -> (-81.4929, 21.1929) centre (-82.2, 20.4858) ccw
  arc A217 (-81.4929, 3.0071) -> (-81.2, 3.7142) centre (-82.2, 3.7142) ccw
  arc A218 (-81.2, -4.3142) -> (-81.4929, -3.6071) centre (-82.2, -4.3142) ccw
  arc A219 (-81.4929, -21.7929) -> (-81.2, -21.0858) centre (-82.2, -21.0858) ccw
  arc A220 (-87.7142, -27.6) -> (-87.0071, -27.3071) centre (-87.7142, -26.6) ccw
  arc A221 (-105.1929, -27.3071) -> (-104.4858, -27.6) centre (-104.4858, -26.6) ccw
  arc A222 (-111, -21.0858) -> (-110.7071, -21.7929) centre (-110, -21.0858) ccw
  arc A223 (-110.7071, -3.6071) -> (-111, -4.3142) centre (-110, -4.3142) ccw
  arc A224 (-111, 3.7142) -> (-110.7071, 3.0071) centre (-110, 3.7142) ccw
  line L504 (-108.8, 23.1) -> (-108.2, 23.1)
  line L505 (-107.1, 0) -> (-107.1, -0.6)
  line L506 (-105.1929, -2.5071) -> (-107.1, -0.6)
  line L507 (-108.8, -1.7) -> (-108.2, -1.7)
  line L508 (-108.8, -23.7) -> (-108.2, -23.7)
  line L509 (-103.9, 20.9) -> (-88.3, 20.9)
  line L510 (-86.2, 20.4858) -> (-86.2, 3.7142)
  line L511 (-88.3, 3.3) -> (-103.9, 3.3)
  line L512 (-106, 3.7142) -> (-106, 20.4858)
  line L513 (-104.4858, 22) -> (-87.7142, 22)
  line L514 (-87.3, 19.9) -> (-87.3, 4.3)
  line L515 (-87.7142, 2.2) -> (-104.4858, 2.2)
  line L516 (-104.9, 4.3) -> (-104.9, 19.9)
  line L517 (-103.9, -3.9) -> (-88.3, -3.9)
  line L518 (-86.2, -4.3142) -> (-86.2, -21.0858)
  line L519 (-88.3, -21.5) -> (-103.9, -21.5)
  line L520 (-106, -21.0858) -> (-106, -4.3142)
  line L521 (-104.4858, -22.6) -> (-87.7142, -22.6)
  line L522 (-87.3, -20.5) -> (-87.3, -4.9)
  line L523 (-87.7142, -2.8) -> (-104.4858, -2.8)
  line L524 (-104.9, -4.9) -> (-104.9, -20.5)
  arc A225 (-85.9071, 21.1929) -> (-86.2, 20.4858) centre (-85.2, 20.4858) ccw
  arc A226 (-87.7142, 22) -> (-87.0071, 22.2929) centre (-87.7142, 23) ccw
  arc A227 (-105.1929, 22.2929) -> (-104.4858, 22) centre (-104.4858, 23) ccw
  arc A228 (-106, 20.4858) -> (-106.2929, 21.1929) centre (-107, 20.4858) ccw
  arc A229 (-86.2, 3.7142) -> (-85.9071, 3.0071) centre (-85.2, 3.7142) ccw
  arc A230 (-85.9071, -3.6071) -> (-86.2, -4.3142) centre (-85.2, -4.3142) ccw
  arc A231 (-87.0071, 1.9071) -> (-87.7142, 2.2) centre (-87.7142, 1.2) ccw
  arc A232 (-87.7142, -2.8) -> (-87.0071, -2.5071) centre (-87.7142, -1.8) ccw
  arc A233 (-105.1929, -2.5071) -> (-104.4858, -2.8) centre (-104.4858, -1.8) ccw
  arc A234 (-104.4858, 2.2) -> (-105.1929, 1.9071) centre (-104.4858, 1.2) ccw
  arc A235 (-106, -4.3142) -> (-106.2929, -3.6071) centre (-107, -4.3142) ccw
  arc A236 (-106.2929, 3.0071) -> (-106, 3.7142) centre (-107, 3.7142) ccw
  arc A237 (-103.9, -3.9) -> (-104.9, -4.9) centre (-103.9, -4.9) ccw
  arc A238 (-87.3, -4.9) -> (-88.3, -3.9) centre (-88.3, -4.9) ccw
  arc A239 (-88.3, -21.5) -> (-87.3, -20.5) centre (-88.3, -20.5) ccw
  arc A240 (-87.0071, -22.8929) -> (-87.7142, -22.6) centre (-87.7142, -23.6) ccw
  arc A241 (-104.9, -20.5) -> (-103.9, -21.5) centre (-103.9, -20.5) ccw
  arc A242 (-106.2929, -21.7929) -> (-106, -21.0858) centre (-107, -21.0858) ccw
  arc A243 (-104.4858, -22.6) -> (-105.1929, -22.8929) centre (-104.4858, -23.6) ccw
  arc A244 (-87.3, 19.9) -> (-88.3, 20.9) centre (-88.3, 19.9) ccw
  arc A245 (-103.9, 20.9) -> (-104.9, 19.9) centre (-103.9, 19.9) ccw
  arc A246 (-88.3, 3.3) -> (-87.3, 4.3) centre (-88.3, 4.3) ccw
  arc A247 (-104.9, 4.3) -> (-103.9, 3.3) centre (-103.9, 4.3) ccw
  arc A248 (-86.2, -21.0858) -> (-85.9071, -21.7929) centre (-85.2, -21.0858) ccw
  line L525 (10.9, 11) -> (11.9, 11)
  line L526 (11.9, 11) -> (13.9, 9)
  line L527 (13.9, 9) -> (13.9, 8)
  line L528 (13.9, 8) -> (11.9, 6)
  line L529 (11.9, 6) -> (10.9, 6)
  line L530 (10.9, 6) -> (8.9, 8)
  line L531 (8.9, 8) -> (8.9, 9)
  line L532 (8.9, 9) -> (10.9, 11)
  line L533 (10.9, -9) -> (11.9, -9)
  line L534 (11.9, -9) -> (13.9, -11)
  line L535 (13.9, -11) -> (13.9, -12)
  line L536 (13.9, -12) -> (11.9, -14)
  line L537 (11.9, -14) -> (10.9, -14)
  line L538 (10.9, -14) -> (8.9, -12)
  line L539 (8.9, -12) -> (8.9, -11)
  line L540 (8.9, -11) -> (10.9, -9)
  line L541 (-73.2, 11) -> (-72.2, 11)
  line L542 (-72.2, 11) -> (-70.2, 9)
  line L543 (-70.2, 9) -> (-70.2, 8)
  line L544 (-70.2, 8) -> (-72.2, 6)
  line L545 (-72.2, 6) -> (-73.2, 6)
  line L546 (-73.2, 6) -> (-75.2, 8)
  line L547 (-75.2, 8) -> (-75.2, 9)
  line L548 (-75.2, 9) -> (-73.2, 11)
  line L549 (-73.2, -9) -> (-72.2, -9)
  line L550 (-72.2, -9) -> (-70.2, -11)
  line L551 (-70.2, -11) -> (-70.2, -12)
  line L552 (-70.2, -12) -> (-72.2, -14)
  line L553 (-72.2, -14) -> (-73.2, -14)
  line L554 (-73.2, -14) -> (-75.2, -12)
  line L555 (-75.2, -12) -> (-75.2, -11)
  line L556 (-75.2, -11) -> (-73.2, -9)
  point P0 (154.8, 18)
  point P1 (143.2, 13)
  point P2 (137.8, 18)
  point P3 (143, 0.1858)
  point P4 (143, 11.7858)
  point P5 (138, 0.1858)
  point P6 (138, -5.2142)
  point P7 (138, -16.8142)
  point P8 (96.7, 2)
  point P9 (96.7, -3)
  point P10 (126.3, 2)
  point P11 (109, 14.3)
  point P12 (114, -15.3)
  point P13 (114, 14.3)
  point P14 (109, -15.3)
  point P15 (154.8, 13)
  point P16 (138, 11.7858)
  point P17 (143, -5.2142)
  point P18 (126.3, -3)
  point P19 (143, -16.8142)
  point P20 (137.8, 13)
  point P21 (126.2, 13)
  point P22 (126.2, 18)
  point P23 (108.3, 2)
  point P24 (114, 2.7)
  point P25 (109, -3.7)
  point P26 (114, -3.7)
  point P27 (109, 2.7)
  point P28 (108.3, -3)
  point P29 (114.7, -3)
  point P30 (114.7, 2)
  point P31 (143.2, 18)
  point P32 (143.2, 18)
  point P33 (126.2, 18)
  point P34 (138, 11.7858)
  point P35 (143, -16.3142)
  point P36 (143, -4.7142)
  point P37 (142.7071, -4.4213)
  point P38 (109.5929, 1.7071)
  point P39 (97.4071, 1.7071)
  point P40 (109.5929, -2.7071)
  point P41 (110.2929, -3.4071)
  point P42 (110.2929, -15.5929)
  point P43 (127.3, -3)
  point P44 (129.5, -0.8)
  point P45 (129.5, -0.2)
  point P46 (115.4071, 1.7071)
  point P47 (114.7071, 2.4071)
  point P48 (114.7071, 14.5929)
  point P49 (-145.5, 23.1)
  point P50 (-146.1, 23.1)
  point P51 (-144.4, 0)
  point P52 (-144.4, -0.6)
  point P53 (-145.5, -1.7)
  point P54 (-146.1, -1.7)
  point P55 (-146.1, -23.7)
  point P56 (-145.5, -23.7)
  point P57 (-108.2, 23.1)
  point P58 (-108.8, 23.1)
  point P59 (-107.1, 0)
  point P60 (-107.1, -0.6)
  point P61 (-108.2, -1.7)
  point P62 (-108.8, -1.7)
  point P63 (-108.8, -23.7)
  point P64 (-108.2, -23.7)
  point P65 (-61.4, 23.1)
  point P66 (-62, 23.1)
  point P67 (-60.3, 0)
  point P68 (-60.3, -0.6)
  point P69 (-61.4, -1.7)
  point P70 (-62, -1.7)
  point P71 (-62, -23.7)
  point P72 (-61.4, -23.7)
  point P73 (-24.1, 23.1)
  point P74 (-24.7, 23.1)
  point P75 (-23, 0)
  point P76 (-23, -0.6)
  point P77 (-24.1, -1.7)
  point P78 (-24.7, -1.7)
  point P79 (-24.7, -23.7)
  point P80 (-24.1, -23.7)
  point P81 (22.7, 23.1)
  point P82 (22.1, 23.1)
  point P83 (23.8, 0)
  point P84 (23.8, -0.6)
  point P85 (22.7, -1.7)
  point P86 (22.1, -1.7)
  point P87 (22.1, -23.7)
  point P88 (22.7, -23.7)
  point P89 (80.4858, 27)
  point P90 (63.7142, 27)
  point P91 (60, 23.1)
  point P92 (59.4, 23.1)
  point P93 (61.1, 0)
  point P94 (61.1, -0.6)
  point P95 (60, -1.7)
  point P96 (59.4, -1.7)
  point P97 (59.4, -23.7)
  point P98 (60, -23.7)
  point P99 (43.6, -2.8)
  point P100 (43.6, 2.2)
  point P101 (26, 2.2)
  point P102 (26, -2.8)
  point P103 (-59.2, 3.3)
  point P104 (-59.2, 20.9)
  point P105 (-106, -21.5)
  point P106 (-106, -3.9)
  point P107 (-143.3, -21.5)
  point P108 (-143.3, -3.9)
  point P109 (-124.6, -2.8)
  point P110 (-124.6, 2.2)
  point P111 (-142.2, 2.2)
  point P112 (-142.2, -2.8)
  point P113 (-87.3, -2.8)
  point P114 (-87.3, 2.2)
  point P115 (-104.9, 2.2)
  point P116 (-104.9, -2.8)
  point P117 (-3.2, -2.8)
  point P118 (-3.2, 2.2)
  point P119 (-20.8, 2.2)
  point P120 (-20.8, -2.8)
  point P121 (80.9, -2.8)
  point P122 (80.9, 2.2)
  point P123 (63.3, 2.2)
  point P124 (63.3, -2.8)
  point P125 (44.7, 20.9)
  point P126 (44.7, 3.3)
  point P127 (-40.5, -2.8)
  point P128 (-40.5, 2.2)
  point P129 (-58.1, 2.2)
  point P130 (-58.1, -2.8)
  point P131 (-39.4, 20.9)
  point P132 (-39.4, 3.3)
  point P133 (-86.2, -21.5)
  point P134 (-86.2, -3.9)
  point P135 (-143.3, 3.3)
  point P136 (-143.3, 20.9)
  point P137 (-142.2, -22.6)
  point P138 (-124.6, -22.6)
  point P139 (-123.5, -21.5)
  point P140 (-123.5, -3.9)
  point P141 (-123.5, 20.9)
  point P142 (-123.5, 3.3)
  point P143 (-142.2, 22)
  point P144 (-124.6, 22)
  point P145 (-106, 3.3)
  point P146 (-106, 20.9)
  point P147 (-104.9, 22)
  point P148 (-87.3, 22)
  point P149 (-86.2, 20.9)
  point P150 (-86.2, 3.3)
  point P151 (-104.9, -22.6)
  point P152 (-87.3, -22.6)
  point P153 (-58.1, -22.6)
  point P154 (-40.5, -22.6)
  point P155 (-59.2, -21.5)
  point P156 (-59.2, -3.9)
  point P157 (-39.4, -21.5)
  point P158 (-39.4, -3.9)
  point P159 (-58.1, 22)
  point P160 (-40.5, 22)
  point P161 (-20.8, -22.6)
  point P162 (-3.2, -22.6)
  point P163 (-21.9, -21.5)
  point P164 (-21.9, -3.9)
  point P165 (-21.9, 3.3)
  point P166 (-21.9, 20.9)
  point P167 (-20.8, 22)
  point P168 (-3.2, 22)
  point P169 (-2.1, 20.9)
  point P170 (-2.1, 3.3)
  point P171 (-2.1, -21.5)
  point P172 (-2.1, -3.9)
  point P173 (24.9, -21.5)
  point P174 (24.9, -3.9)
  point P175 (26, 22)
  point P176 (43.6, 22)
  point P177 (24.9, 3.3)
  point P178 (24.9, 20.9)
  point P179 (44.7, -21.5)
  point P180 (44.7, -3.9)
  point P181 (26, -22.6)
  point P182 (43.6, -22.6)
  point P183 (63.3, -22.6)
  point P184 (80.9, -22.6)
  point P185 (82, -21.5)
  point P186 (82, -3.9)
  point P187 (62.2, -21.5)
  point P188 (62.2, -3.9)
  point P189 (62.2, 3.3)
  point P190 (62.2, 20.9)
  point P191 (63.3, 22)
  point P192 (80.9, 22)
  point P193 (82, 20.9)
  point P194 (82, 3.3)
  dimension "d1264" = 0
  dimension "d1265" = 0
  dimension "d1266" = 0
  dimension "d1267" = 0
  dimension "d1268" = 0
  dimension "d1269" = 0
  dimension "d1270" = 0
  dimension "d1271" = 0
  dimension "d1272" = 0
  dimension "d1273" = 0
  dimension "d1274" = 0
  dimension "d1275" = 0
  dimension "d1276" = 0
  dimension "d1277" = 0
  dimension "d1278" = 0
  dimension "d1279" = 0
  dimension "d1280" = 0
  dimension "d1281" = 0
  dimension "d1282" = 0
  dimension "d1283" = 0
  dimension "d1308" = 1
  dimension "d1309" = 1
  dimension "d1310" = 1
  dimension "d1311" = 1
  dimension "d1312" = 1
  dimension "d1313" = 1
  constraints: 154 end point, 83 point on line, 66 point on circle, 66 tangent, 33 centre point, 27 equal radius, 26 parallel, 18 collinear, 13 perpendicular, 8 horizontal, 3 vertical
  measures "d1264" vertical extent of L97
  measures "d1265" vertical extent of L98
  measures "d1266" vertical extent of L99
  measures "d1267" vertical extent of L100
  measures "d1268" vertical extent of L101
  measures "d1269" vertical extent of L102
  measures "d1270" horizontal extent of L103
  measures "d1271" horizontal extent of L104